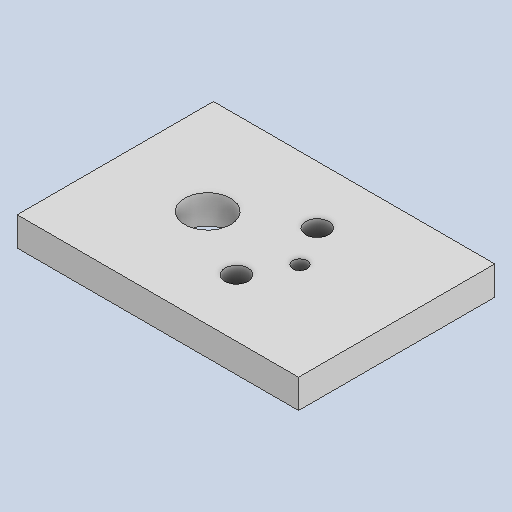
# Autodesk Inventor part: AR-BracketRight2
Saved by Autodesk Inventor 2025.1 (Build 291241020, 241B)
## iProperties
Created: 2025-05-09
Part Number: AR-BracketRight2
Material: Generic
Document SubType Name: Modeling
Designer: t205b
Density: 1 g/cm^3
Appearance: Default
Author: t205b
Autodesk Inventor part; units mm, degrees
ref_plane "YZ Plane" through (0, 0, 0) normal (1, 0, 0) x (0, 1, 0)
ref_plane "XZ Plane" through (0, 0, 0) normal (0, 1, 0) x (-1, 0, 0)
ref_plane "XY Plane" through (0, 0, 0) normal (0, 0, 1) x (1, 0, 0)
sketch "Sketch1" plane through (0, 0, 0) normal (0, 1, 0) x (-1, 0, 0)
  line L0 (0, 0) -> (61.9125, 0)
  line L1 (61.9125, 0) -> (61.9125, -43.18)
  line L2 (61.9125, -43.18) -> (0, -43.18)
  line L3 (0, -43.18) -> (0, 0)
  dimension "d0" = 61.9125
  dimension "d1" = 43.18
  constraints: 8 end point, 2 parallel, 1 horizontal, 1 perpendicular
  measures "d0" distance between parallel lines of L3 L1
  measures "d1" distance between parallel lines of L0 L2
extrude "Extrusion1" add sketch "Sketch1" along normal blind 6.35
sketch "Sketch2" plane through (0, 6.35, 0) normal (0, 1, 0) x (1, 0, 0)
  line L0 (-61.9125, 43.18) -> (-61.9125, 0)
  line L1 (-61.9125, 0) -> (0, 0)
  line L2 (0, 0) -> (0, 43.18)
  line L3 (-61.9125, 43.18) -> (0, 43.18)
  line L4 (-61.9125, 43.18) -> (-61.9125, 0) projected
  line L5 (0, 43.18) -> (-61.9125, 43.18) projected
  line L6 (-61.9125, 0) -> (0, 0) projected
  line L7 (0, 0) -> (0, 43.18) projected
  point P0 (-41.5925, 21.59)
  point P1 (-21.2725, 21.59)
  point P2 (-26.3525, 30.48)
  point P3 (-26.3525, 12.7)
  dimension "d10" = 21.2725
  dimension "d11" = 21.59
  dimension "d14" = 21.59
  dimension "d15" = 20.32
  dimension "d18" = 12.7
  dimension "d19" = 12.7
  dimension "d20" = 15.24
  dimension "d21" = 15.24
  constraints: 8 end point, 4 collinear
  measures "d10" distance from line of L2 point (-21.272, 21.59)
  measures "d11" distance from line of L1 point (-21.272, 21.59)
  measures "d14" distance from line of L1 point (-41.593, 21.59)
  measures "d15" distance from line of L0 point (-41.593, 21.59)
  measures "d18" distance from line of L1 point (-26.353, 12.7)
  measures "d19" distance from line of L3 point (-26.353, 30.48)
  measures "d20" horizontal distance of point (-26.353, 12.7) point (-41.593, 21.59)
  measures "d21" horizontal distance of point (-41.593, 21.59) point (-26.353, 30.48)
hole "Hole1" at (-21.2725, 6.35, -21.59) direction (0, -1, 0) diameter 3.175 depth 10.9728 tip angle 118
hole "Hole2" at (-41.5925, 6.35, -21.59) direction (0, -1, 0) diameter 10.1001 end through all
hole "Hole3" at (-26.3525, 6.35, -30.48) at (-26.3525, 6.35, -12.7) direction (0, -1, 0) diameter 5.1054 end through all clearance for "Flat Head Machine Screw (82)" size "#10" standard "Ansi Unified Screw Threads"
sketch "Sketch3" plane through (-61.9125, 0, -43.18) normal (-1, 0, 0) x (0, 0, 1)
  line L0 (43.18, 0) -> (43.18, 6.35) projected
  line L1 (0, 0) -> (0, 6.35) projected
  line L2 (0, 0) -> (43.18, 0) projected
  point P0 (6.35, 3.175)
  point P1 (36.83, 3.175)
  dimension "d50" = 6.35
  dimension "d51" = 6.35
  dimension "d52" = 3.175
  constraints: 1 horizontal alignment
  measures "d50" distance from line of L0 point (36.83, 3.175)
  measures "d51" distance from line of L1 point (6.35, 3.175)
  measures "d52" distance from line of point (6.35, 3.175) L2
hole "Hole4" at (-61.9125, 3.175, -36.83) at (-61.9125, 3.175, -6.35) direction (1, 0, 0) diameter 2.6416 depth 10.9728 tip angle 118 thread size "6-32 UNC" class "3B" standard "ANSI Unified Screw Threads"
body "Solid1"
